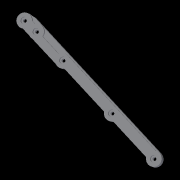
# Autodesk Inventor part: ShinLockLeft
Saved by Autodesk Inventor 2015 SP1 (Build 190203100, 203)
## iProperties
RuleStatus: InUse
Created: 2014-12-04
Part Number: ShinLockLeft
Material: Generic
Document SubType Name: Modeling
Designer: Val
Density: 1 g/cm^3
Appearance: Default
Mass: 119.144 g
Surface Area: 469.889 cm^2
Volume: 119.144 cm^3
BeforeDocSave0: UpdateBoundingBox
CX: 27.00 mm
CY: 325.00 mm
CZ: 10.50 mm
Author: Val
Autodesk Inventor part; units mm, degrees
ref_plane "YZ Plane" through (0, 0, 0) normal (1, 0, 0) x (0, 1, 0)
ref_plane "XZ Plane" through (0, 0, 0) normal (0, 1, 0) x (-1, 0, 0)
ref_plane "XY Plane" through (0, 0, 0) normal (0, 0, 1) x (1, 0, 0)
sketch "Base" plane through (0, 0, 0) normal (0, 0, 1) x (1, 0, 0)
  circle A0 centre (0, 0) radius 3
  circle A1 centre (0, 0) radius 5.75
  circle A2 centre (0, 0) radius 12.5
  line L0 (0, 0) -> (0, -98) construction
  circle A3 centre (0, -98) radius 3
  circle A4 centre (0, -98) radius 5.75
  arc A5 (10.5, -91.2177) -> (10.5, -104.7823) centre (0, -98) ccw
  line L1 (0, -98) -> (0, -212) construction
  circle A6 centre (0, -212) radius 12.5 construction
  circle A7 centre (0, -212) radius 5.75
  circle A8 centre (0, -212) radius 3
  line L2 (0, -212) -> (0, -274) construction
  circle A9 centre (0, -274) radius 12.5
  circle A10 centre (0, -274) radius 5.75
  circle A11 centre (0, -274) radius 3
  line L3 (0, -274) -> (0, -300) construction
  circle A12 centre (-2, -300) radius 12.5
  circle A13 centre (-2, -300) radius 5.75
  circle A14 centre (-2, -300) radius 3
  line L4 (-7, -10.3562) -> (-7, -87.6438)
  line L5 (-7, -108.3562) -> (-7, -201.6438)
  line L6 (-10.5, -218.7823) -> (-10.5, -267.2177)
  line L7 (-10.5, -280.7823) -> (-10.5, -290.8348)
  line L8 (-12.5, -212) -> (-12.5, -274) construction
  line L9 (12.5, 0) -> (12.5, -212) construction
  line L10 (10.5, -6.7823) -> (10.5, -91.2177)
  line L11 (10.5, -104.7823) -> (10.5, -205.2177)
  line L12 (2, -224.339) -> (2, -261.661)
  line L13 (6.5, -284.6771) -> (6.5, -290.8348)
  line L14 (10.5, -104.7823) -> (10.5, -91.2177)
  line L15 (10.5, -205.2177) -> (10.5, -214.3503)
  arc A15 (2, -224.339) -> (10.5, -214.3503) centre (0.381, -214.3503) ccw
  arc A16 (-7, -201.6438) -> (-10.5, -218.7823) centre (0, -212) ccw
  line L16 (0, -300) -> (-2, -300) construction
  dimension "d401" = 6
  dimension "d404" = 11.5
  dimension "d405" = 25
  dimension "d406" = 98
  dimension "d407" = 114
  dimension "d408" = 62
  dimension "d409" = 26
  dimension "d412" = 7
  dimension "d414" = 2
  dimension "d415" = 2
  dimension "d416" = 2
  dimension "d421" = 17
  dimension "d427" = 2
  constraints: 34 end point, 25 point on circle, 17 centre point, 15 coincident, 11 equal radius, 9 vertical, 5 parallel, 5 tangent, 3 collinear, 1 horizontal
  measures "d401" diameter of A0
  measures "d404" diameter of A1
  measures "d405" diameter of A2
  measures "d406" distance of L0.start L0.end
  measures "d407" distance of L1.start L1.end
  measures "d408" distance of L2.start L2.end
  measures "d409" distance of L3.start L3.end
  measures "d412" distance between parallel lines of L4 L0
  measures "d414" distance between parallel lines of L8 L6
  measures "d415" distance between parallel lines of L9 L10
  measures "d416" distance between parallel lines of L12 L2
  measures "d421" distance between parallel lines of L13 L7
  measures "d427" distance of L3.end L16.end
extrude "BaseFeature" add sketch "Base" along normal blind 3.5 contours A2 | A2 L10 A5 L4 | A5 L14 | A5 L11 L15 A15 L12 A9 L6 A16 L5 | A9 | A9 L13 A12 L7 | A12
sketch "Mount" plane through (0, 0, 0) normal (0, 0, -1) x (-1, 0, 0)
  line L0 (12.2472, -209.4989) -> (12.5759, -293.3366)
  arc A0 (-6.5, -290.8348) -> (10.5, -290.8348) centre (2, -300) ccw projected
  line L1 (-12.5, -292.0568) -> (-10.4919, -299.551)
  line L2 (7, -10.3562) -> (7, -87.6438) projected
  arc A1 (7, -108.3562) -> (7, -87.6438) centre (0, -98) ccw projected
  circle A2 centre (0, 0) radius 3 projected
  circle A3 centre (0, -98) radius 3 projected
  circle A4 centre (0, -212) radius 3 projected
  circle A5 centre (0, -274) radius 3 projected
  circle A6 centre (2, -300) radius 3 projected
  arc A7 (10.5, -218.7823) -> (7, -201.6438) centre (0, -212) ccw projected
  line L3 (7, -108.3562) -> (7, -201.6438) projected
  line L4 (-12.5, -292.0568) -> (-12.5, 0)
  line L5 (-10.5, -214.3503) -> (-10.5, -6.7823) construction
  arc A8 (-6.5, -290.8348) -> (10.5, -290.8348) centre (2, -300) ccw projected
  arc A9 (7, -10.3562) -> (-10.5, -6.7823) centre (0, 0) ccw projected
  arc A10 (10.5, -280.7823) -> (10.5, -267.2177) centre (0, -274) ccw projected
  arc A11 (-2, -261.661) -> (-6.5, -284.6771) centre (0, -274) ccw projected
  line L6 (-12.5, -292.0568) -> (12.5705, -291.9585) construction
  dimension "d430" = 8
  dimension "d431" = 165
  constraints: 8 end point, 5 point on circle, 2 tangent, 1 perpendicular, 1 point on line, 1 vertical
  measures "d430" distance from line of A0.centre L6
  measures "d431" angle of L4 L1
extrude "MountFeature" add sketch "Mount" along normal blind 7 contours L0 A0 L1 L4 A9 L2 A1 L3 A7
mirror "LeftMirrorFeature" about plane through (0, 0, 0) normal (1, 0, 0) remove original yes
